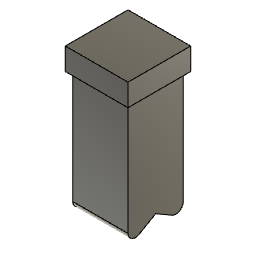
Clamp Bar Short v1 (Autodesk Fusion 360 design; units mm, degrees)
Autodesk Fusion 360 part; units mm, degrees
sketch "Sketch1" plane through (0, 0, 0) normal (0, 0, 1) x (1, 0, 0)
  line L0 (0, 0) -> (8.5, 0)
  line L1 (8.5, 0) -> (8.5, 8.5)
  line L2 (8.5, 8.5) -> (0, 8.5)
  line L3 (0, 8.5) -> (0, 0)
  dimension "d1" = 8.5
  constraint horizontal L0
  constraint vertical L1
  constraint horizontal L2
  constraint vertical L3
  constraint coincident L0.start L3.end
  constraint equal L1 L2
  measures "d1" distance of L0.end L1.end
extrude "Extrude1" add sketch "Sketch1" along normal blind 3
sketch "Sketch2" plane through (0, 0, 0) normal (0, 0, -1) x (1, 0, 0)
  line L0 (0, 0) -> (0, -8.5)
  line L1 (0, -8.5) -> (8.5, -8.5)
  line L2 (8.5, -8.5) -> (8.5, 0)
  line L3 (8.5, 0) -> (0, 0)
  line L4 (0.5, -0.5) -> (8, -0.5)
  line L5 (8, -0.5) -> (8, -8)
  line L6 (8, -8) -> (0.5, -8)
  line L7 (0.5, -8) -> (0.5, -0.5)
  line L8 (0.5, -0.5) -> (8, -8) construction
  line L9 (8.5, 0) -> (0, -8.5) construction
  dimension "d4" = 7.5
  constraint horizontal L4
  constraint vertical L5
  constraint horizontal L6
  constraint vertical L7
  constraint coincident L2.end L3.start
  constraint coincident L0.end L1.start
  constraint midpoint L8 L9
  constraint equal L4 L7
  measures "d4" distance of L4.start L4.end
extrude "Extrude2" add sketch "Sketch2" along normal blind 17 contours L4 L5 L6 L7
sketch "Sketch3" plane through (8, 0, 0) normal (1, 0, 0) x (0, 1, 0)
  line L0 (8, 0) -> (0.5, 0)
  line L1 (0.5, 0) -> (0.5, -17)
  line L2 (0.5, -17) -> (8, -17)
  line L3 (8, -17) -> (8, 0)
  line L4 (0.5, -17) -> (4.25, -14.8349)
  line L5 (4.25, -14.8349) -> (8, -17)
  line L6 (8, -17) -> (0.5, -17)
  dimension "d7" = 120
  constraint coincident L1.end L2.start
  constraint coincident L2.end L3.start
  constraint equal L4 L5
  measures "d7" angle of L4 L5
extrude "Extrude3" cut sketch "Sketch3" against normal through all contours L2 L4 L5 L6
fillet "Fillet1" radius 1 2 edges at (4.25, 0.5, -17) (4.25, 8, -17)
